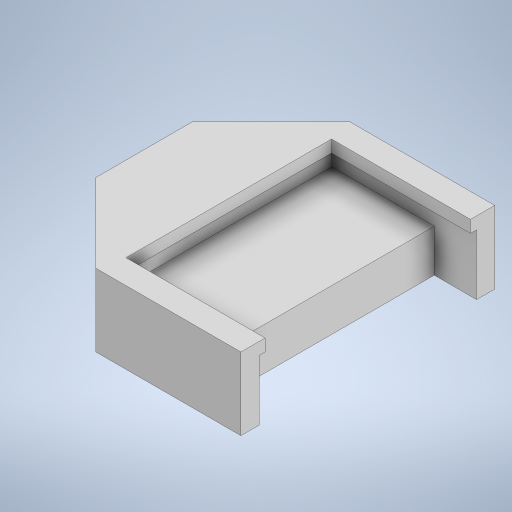
# Autodesk Inventor part: sensorHolder
Saved by Autodesk Inventor 2023.1 (Build 271208000, 208)
## iProperties
Created: 2024-03-17
Part Number: sensorHolder
Material: Generic
Document SubType Name: Modeling
Designer: Y9650
Density: 1 g/cm^3
Appearance: Default
Author: Y9650
Autodesk Inventor part; units mm, degrees
ref_plane "YZ Plane" through (0, 0, 0) normal (1, 0, 0) x (0, 1, 0)
ref_plane "XZ Plane" through (0, 0, 0) normal (0, 1, 0) x (-1, 0, 0)
ref_plane "XY Plane" through (0, 0, 0) normal (0, 0, 1) x (1, 0, 0)
sketch "Sketch1" plane through (0, 0, 0) normal (0, 1, 0) x (-1, 0, 0)
  line L0 (0, 0) -> (-12, 0)
  line L1 (-12, 0) -> (-12, -17)
  line L2 (-12, -17) -> (0, -17)
  line L3 (0, -17) -> (0, 0)
  line L4 (0, 0) -> (2, 0)
  line L5 (2, 0) -> (2, 2)
  line L6 (2, 2) -> (-12, 2)
  line L7 (-12, 2) -> (-12, -19)
  line L8 (-12, -19) -> (2, -19)
  line L9 (2, -19) -> (2, 2)
  dimension "d0" = 12
  dimension "d1" = 17
  dimension "d2" = 2
  dimension "d3" = 2
  dimension "d4" = 21
  constraints: 20 end point, 4 parallel, 3 horizontal, 3 perpendicular
  measures "d0" distance of L2.end L1.end
  measures "d1" distance of L1.end L0.end
  measures "d2" distance of L0.start L4.end
  measures "d3" distance of L4.end L5.end
  measures "d4" distance of L7.end L6.end
extrude "Extrusion1" add sketch "Sketch1" along normal blind 4
sketch "Sketch3" plane through (0, 4, 0) normal (0, 1, 0) x (1, 0, 0)
  line L0 (12, -2) -> (12, 19) projected
  line L1 (0, 0) -> (12, 0)
  line L2 (12, 0) -> (12, 17)
  line L3 (12, 17) -> (0, 17)
  line L4 (0, 17) -> (0, 0)
  dimension "d7" = 17
  constraints: 8 end point, 2 parallel, 1 horizontal, 1 perpendicular, 1 point on line
  measures "d7" distance of L2.end L1.end
extrude "Extrusion2" cut sketch "Sketch3" against normal blind 2.5
sketch "Sketch4" plane through (0, 4, 0) normal (1, 0, 0) x (0, 0, -1)
  line L0 (-2, 0) -> (0, 0) projected
  line L1 (17, 0) -> (17, -2.5) projected
  line L2 (0, 0) -> (17, 0)
  line L3 (17, 0) -> (17, -1.5)
  line L4 (17, -1.5) -> (0, -1.5)
  line L5 (0, -1.5) -> (0, 0)
  point P0 (0, -4)
  dimension "d10" = 1.5
  constraints: 8 end point, 2 parallel, 1 horizontal, 1 perpendicular, 1 point on line
  measures "d10" distance of L2.end L3.end
extrude "Extrusion3" add sketch "Sketch4" along normal blind 0.5
sketch "Sketch5" plane through (0, 1.5, -17) normal (0, 0, 1) x (1, 0, 0)
  line L0 (12, 2.5) -> (12, 0) projected
  line L1 (0.5, 2.5) -> (12, 2.5)
  line L2 (12, 2.5) -> (12, 1)
  line L3 (12, 1) -> (0.5, 1)
  line L4 (0.5, 1) -> (0.5, 2.5)
  point P0 (0, -1.5)
  dimension "d13" = 1.5
  constraints: 8 end point, 2 parallel, 1 horizontal, 1 perpendicular, 1 point on line
  measures "d13" distance of L1.end L2.end
extrude "Extrusion4" add sketch "Sketch5" along normal blind 0.5
sketch "Sketch6" plane through (12, 1.5, 0) normal (0, 0, -1) x (-1, 0, 0)
  line L0 (14, 2.5) -> (0, 2.5) projected
  line L1 (12, 1) -> (11.5, 1) projected
  line L2 (0, 2.5) -> (11.5, 2.5)
  line L3 (11.5, 2.5) -> (11.5, 1)
  line L4 (11.5, 1) -> (0, 1)
  line L5 (0, 1) -> (0, 2.5)
  point P0 (12, -1.5)
  dimension "d20" = 1.5
  constraints: 8 end point, 2 parallel, 1 horizontal, 1 perpendicular
  measures "d20" distance of L4.end L0.end
extrude "Extrusion5" add sketch "Sketch6" along normal blind 0.5
sketch "Sketch7" plane through (12, 0, 2) normal (1, 0, 0) x (0, 0, -1)
  line L0 (19, 2.5) -> (19, 1.5) projected
  line L1 (19, 1.5) -> (2, 1.5)
  line L2 (2, 1.5) -> (2, 0)
  line L3 (2, 0) -> (19, 0)
  line L4 (19, 0) -> (19, 1.5)
  constraints: 8 end point, 2 parallel, 1 horizontal, 1 perpendicular
extrude "Extrusion6" cut sketch "Sketch7" against normal blind 3.5
sketch "Sketch8" plane through (-2, 0, -19) normal (-1, 0, 0) x (0, 0, 1)
  line L0 (0, 0) -> (21, 0) projected
  line L1 (21, 0) -> (21, 4) projected
  line L2 (0, 4) -> (21, 4) projected
  line L3 (0, 0) -> (0, 4) projected
  point P0 (19, 0)
extrude "Extrusion7" add sketch "Sketch8" along normal blind 4.5
chamfer "Chamfer2" distance 6.5 angle 45 1 edges at (-6.5, 2, 2)
sketch "Sketch16" plane through (0, 2.5, -17) normal (0, 0, 1) x (1, 0, 0)
  line L0 (12, 0) -> (0, 0) projected
  line L1 (0, 0) -> (0, -1) projected
  line L2 (0, -1) -> (8.5, -1) projected
  line L3 (8.5, -1) -> (8.5, -2.5) projected
  line L4 (12, -2.5) -> (8.5, -2.5) projected
  line L5 (12, 0) -> (12, -2.5) projected
  point P0 (0, -2.5)
extrude "Extrusion14" cut sketch "Sketch16" against normal blind 0.5
sketch "Sketch17" plane through (12, 2.5, 0) normal (0, 0, -1) x (-1, 0, 0)
  line L0 (12, 0) -> (0, 0) projected
  line L1 (0, -2.5) -> (0, 0) projected
  line L2 (3.5, -2.5) -> (0, -2.5) projected
  line L3 (3.5, -2.5) -> (3.5, -1) projected
  line L4 (3.5, -1) -> (12, -1) projected
  line L5 (12, 0) -> (12, -1) projected
  point P0 (12, -2.5)
extrude "Extrusion15" cut sketch "Sketch17" against normal blind 0.5
sketch "Sketch18" plane through (0.5, 2.5, -16.5) normal (0, -1, 0) x (1, 0, 0)
  line L0 (-0.5, -1) -> (-0.5, 17) projected
  line L1 (-0.5, -1) -> (11.5, -1) projected
  line L2 (11.5, 0) -> (11.5, -1) projected
  line L3 (0, 0) -> (11.5, 0) projected
  line L4 (0, 16) -> (0, 0) projected
  line L5 (11.5, 16) -> (0, 16) projected
  line L6 (11.5, 17) -> (11.5, 16) projected
  line L7 (11.5, 17) -> (-0.5, 17) projected
  point P0 (-0.5, 16.5)
extrude "Extrusion16" cut sketch "Sketch18" against normal blind 0.5
chamfer "Chamfer3" distance 6.5 angle 45 1 edges at (-6.5, 2, -19)
sketch "Sketch19" plane through (0, 0, 0) normal (0, -1, 0) x (1, 0, 0)
  line L0 (0, -19) -> (-6.5, -12.5) projected
  line L1 (12, -19) -> (0, -19) projected
  line L2 (12, -17.5) -> (12, -19) projected
  line L3 (12, -17.5) -> (8.5, -17.5) projected
  line L4 (8.5, -17.5) -> (8.5, 0.5) projected
  line L5 (8.5, 0.5) -> (12, 0.5) projected
  line L6 (12, 2) -> (12, 0.5) projected
  line L7 (12, 2) -> (0, 2) projected
  line L8 (-6.5, -4.5) -> (0, 2) projected
  line L9 (-6.5, -12.5) -> (-6.5, -4.5) projected
  point P0 (0, 0)
extrude "Extrusion17" add sketch "Sketch19" along normal blind 2
sketch "Sketch22" plane through (0, 1.5, -16.5) normal (0, 0, 1) x (1, 0, 0)
  line L0 (0.5, 1.5) -> (12, 1.5) projected
  line L1 (12, 1.5) -> (12, 2.5) projected
  line L2 (12, 2.5) -> (0.5, 2.5) projected
  line L3 (0.5, 1.5) -> (0.5, 2.5) projected
  point P0 (0, -1.5)
extrude "Extrusion20" cut sketch "Sketch22" against normal blind 0.5
sketch "Sketch23" plane through (12, 1.5, -0.5) normal (0, 0, -1) x (-1, 0, 0)
  line L0 (0, 1.5) -> (11.5, 1.5) projected
  line L1 (11.5, 2.5) -> (11.5, 1.5) projected
  line L2 (11.5, 2.5) -> (0, 2.5) projected
  line L3 (0, 2.5) -> (0, 1.5) projected
  point P0 (12, -1.5)
extrude "Extrusion21" cut sketch "Sketch23" against normal blind 0.5
sketch "Sketch24" plane through (-6.5, 0, -19) normal (-1, 0, 0) x (0, 0, 1)
  circle A0 centre (10.5, 1) radius 2.6
  point P0 (19, 0)
  dimension "d79" = 5.2
  constraints: 1 centre point
  measures "d79" diameter of A0
extrude "Extrusion22" cut sketch "Sketch24" against normal blind 5
sketch "Sketch25" plane through (-1.5, 1, -8.5) normal (-1, 0, 0) x (0, 0, 1)
  circle A0 centre (0, 0) radius 2.6 projected
  line L0 (0, 0) -> (0, -1.5)
  line L1 (0, -1.5) -> (2.1237, -1.5)
  line L2 (0, -1.5) -> (-2.1237, -1.5)
  arc A1 (-2.1237, -1.5) -> (2.1237, -1.5) centre (0, 0) ccw
  arc A2 (2.0494, 1.6) -> (-2.0494, 1.6) centre (0, 0) ccw
  line L3 (0, 0) -> (0, 1.5)
  line L4 (2.1237, 1.5) -> (-2.1237, 1.5)
  line L5 (-2.6, 0) -> (2.6, 0)
  point P0 (8.5, -1)
  dimension "d88" = 1.5
  dimension "d89" = 1.5
  dimension "d90" = 5.2
  constraints: 12 end point, 4 point on circle, 2 centre point, 1 horizontal, 1 perpendicular, 1 point on line, 1 vertical, 11 other
  measures "d88" distance between parallel lines of L5 L1
  measures "d89" distance between parallel lines of L5 L4
  measures "d90" distance of L5.start L5.end
extrude "Extrusion23" add sketch "Sketch25" along normal blind 5 contours L4 A0 | A0 L2 L1
body "Solid1"
